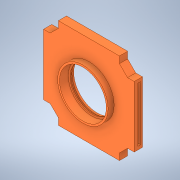
# Autodesk Inventor part: polarbox_20_Lens_holder 1st design
Saved by Autodesk Inventor 2022 (Build 260153000, 153)
## iProperties
Created: 2019-10-23
Part Number: polarbox_20_Lens_holder 1st design
Material: Generic
Document SubType Name: Modeling
Designer: marsikovabarbora
Density: 1 g/cm^3
Appearance: Default
Lens_diameter: 25,000 mm
Author: marsikovabarbora
Autodesk Inventor part; units mm, degrees
ref_plane "YZ Plane" through (0, 0, 0) normal (1, 0, 0) x (0, 1, 0)
ref_plane "XZ Plane" through (0, 0, 0) normal (0, 1, 0) x (-1, 0, 0)
ref_plane "XY Plane" through (0, 0, 0) normal (0, 0, 1) x (1, 0, 0)
sketch "Sketch1" plane through (0, 0, 0) normal (0, 0, 1) x (1, 0, 0)
  line L0 (-34.8609, 0) -> (34.8609, 0) construction
  line L1 (0, -34.8609) -> (0, 34.8609) construction
  line L2 (0, 0) -> (13.4339, 13.4339) construction
  line L3 (0, 0) -> (18.9985, 0) construction
  line L4 (0, 24.9006) -> (16.8, 24.9006)
  line L5 (16.8, 24.9006) -> (16.8, 21.2406)
  line L6 (16.8, 21.2406) -> (19.0203, 19.0203)
  line L7 (24.9006, 0) -> (24.9006, 16.8)
  line L8 (24.9006, 16.8) -> (21.2406, 16.8)
  line L9 (21.2406, 16.8) -> (19.0203, 19.0203)
  line L10 (0, 0) -> (-13.4339, 13.4339) construction
  line L11 (0, 0) -> (-18.9985, 0) construction
  line L12 (0, 24.9006) -> (-16.8, 24.9006)
  line L13 (-16.8, 24.9006) -> (-16.8, 21.2406)
  line L14 (-16.8, 21.2406) -> (-19.0203, 19.0203)
  line L15 (-24.9006, 0) -> (-24.9006, 16.8)
  line L16 (-24.9006, 16.8) -> (-21.2406, 16.8)
  line L17 (-21.2406, 16.8) -> (-19.0203, 19.0203)
  line L18 (0, 0) -> (13.4339, -13.4339) construction
  line L19 (0, -24.9006) -> (16.8, -24.9006)
  line L20 (16.8, -24.9006) -> (16.8, -21.2406)
  line L21 (16.8, -21.2406) -> (19.0203, -19.0203)
  line L22 (24.9006, 0) -> (24.9006, -16.8)
  line L23 (24.9006, -16.8) -> (21.2406, -16.8)
  line L24 (21.2406, -16.8) -> (19.0203, -19.0203)
  line L25 (0, 0) -> (-13.4339, -13.4339) construction
  line L26 (0, -24.9006) -> (-16.8, -24.9006)
  line L27 (-16.8, -24.9006) -> (-16.8, -21.2406)
  line L28 (-16.8, -21.2406) -> (-19.0203, -19.0203)
  line L29 (-24.9006, 0) -> (-24.9006, -16.8)
  line L30 (-24.9006, -16.8) -> (-21.2406, -16.8)
  line L31 (-21.2406, -16.8) -> (-19.0203, -19.0203)
  dimension "d0" = 45
  dimension "d1" = 3.14
  dimension "d2" = 3.66
  dimension "d3" = 16.8
  constraints: 60 end point, 24 symmetric about line, 5 point on line, 2 horizontal, 2 perpendicular, 1 equal length
  measures "d0" angle of L3 L2
  measures "d1" distance of L5.end L6.end
  measures "d2" distance of L4.end L5.end
  measures "d3" distance of L4.start L4.end
extrude "Extrusion1" add sketch "Sketch1" along normal blind 2 and the other way blind 2.5
hole "Hole1" at (0, 0, 0) direction (0, 0, 1) diameter 25.7 end through all both
sketch "Skizze3" plane through (24.9006, -16.8, 2) normal (1, 0, 0) x (0, 0, -1)
  line L0 (0, 33.6) -> (4.5, 33.6) projected
  line L1 (4.5, -4.4406) -> (4.5, 0) projected
  line L2 (2, 33.6) -> (4.5, 33.6) construction
  line L3 (2.7, 33.6) -> (2.7, 0) construction
  line L4 (2, 2.8) -> (2, 36.4349) construction
  line L5 (4.5, 33.6) -> (4.5, 0) construction
  line L6 (0, 0) -> (4.5, 0) projected
  line L7 (2, 31.8) -> (3.5, 31.8)
  line L8 (3.5, 31.8) -> (3.5, 1.8)
  line L9 (3.5, 1.8) -> (2, 1.8)
  line L10 (2, 1.8) -> (2, 31.8)
  point P0 (2, 16.8)
  point P1 (3.5, 16.8)
  point P2 (2.7, 16.8)
  point P3 (2, 16.8)
  point P4 (4.5, 16.8)
  dimension "d25" = 30
  dimension "d26" = 1.5
  dimension "d51" = 1
  constraints: 14 end point, 3 horizontal alignment, 3 midpoint, 3 parallel, 2 horizontal, 2 perpendicular, 3 other
  measures "d25" distance from line of L7 L8.end
  measures "d26" distance between parallel lines of L4 L8
extrude "Extrusion3" cut sketch "Skizze3" against normal up to surface (49.8013 mm away)
sketch "Skizze4" plane through (24.9006, -15, 0) normal (0, 0, -1) x (-1, 0, 0)
  circle A0 centre (24.9006, 15) radius 11.85
  circle A1 centre (24.9006, 15) radius 12.85 projected
  dimension "d33" = 23.7
  dimension "d34" = 1
  constraints: 1 centre point, 1 coincident
  measures "d33" diameter of A0
  measures "d34" radial gap between concentric circles of A1 A0
extrude "Extrusion4" add sketch "Skizze4" against normal blind 0.5
sketch "Sketch7" plane through (0, 0, 2) normal (0, 0, 1) x (1, 0, 0)
  circle A0 centre (0, 0) radius 12.85 construction
  circle A1 centre (0, 0) radius 12.85
  circle A2 centre (0, 0) radius 13.85
  dimension "d52" = 25.7
  dimension "d53" = 1
  constraints: 2 centre point, 2 coincident, 1 concentric
  measures "d52" diameter of A0
  measures "d53" radial gap between concentric circles of A2 A0
extrude "Extrusion7" add sketch "Sketch7" along normal blind 3.3
equation "\"Lens_diameter\" = 25"
body "Solid1"
